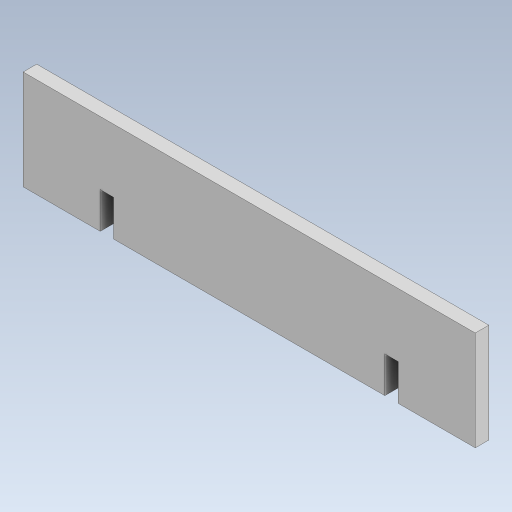
# Autodesk Inventor part: 零件8
Saved by Autodesk Inventor 2023 (Build 270158000, 158)
## iProperties
Created: 2023-05-16
Part Number: 零件8
Material: 一般
Document SubType Name: Modeling
Designer: Johnny Jou
Density: 1 g/cm^3
Appearance: 預設
Author: Johnny Jou
Autodesk Inventor part; units mm, degrees
ref_plane "YZ Plane" through (0, 0, 0) normal (1, 0, 0) x (0, 1, 0)
ref_plane "XZ Plane" through (0, 0, 0) normal (0, 1, 0) x (-1, 0, 0)
ref_plane "XY Plane" through (0, 0, 0) normal (0, 0, 1) x (1, 0, 0)
sketch "草圖1" plane through (0, 0, 0) normal (0, 0, 1) x (1, 0, 0)
  line L0 (0, 0) -> (100, 0)
  line L1 (100, 0) -> (100, -22)
  line L2 (100, -22) -> (0, -22)
  line L3 (0, -22) -> (0, 0)
  line L4 (17.05, -22) -> (20, -22)
  line L5 (20, -22) -> (20, -14)
  line L6 (20, -14) -> (17.05, -14)
  line L7 (17.05, -14) -> (17.05, -22)
  line L8 (80, -22) -> (82.95, -22)
  line L9 (82.95, -22) -> (82.95, -14)
  line L10 (82.95, -14) -> (80, -14)
  line L11 (80, -14) -> (80, -22)
  line L12 (20, -14) -> (80, -14)
  point P0 (50, -14)
  point P1 (50, -22)
  dimension "d0" = 60
  dimension "d1" = 100
  dimension "d2" = 2.95
  dimension "d3" = 2.95
  dimension "d4" = 8
  dimension "d5" = 22
  constraints: 26 end point, 6 parallel, 4 perpendicular, 4 point on line, 2 midpoint, 1 horizontal, 1 vertical alignment
  measures "d0" distance between parallel lines of L11 L5
  measures "d1" distance of L1.end L2.end
  measures "d2" distance of L9.end L10.end
  measures "d3" distance of L5.end L6.end
  measures "d4" distance of L6.end L4.start
  measures "d5" distance of L0.end L1.end
extrude "擠出1" add sketch "草圖1" along normal blind 3 contours L0 L1 L2 L9 L10 L12 L6 L7 L3 | L5 L12 L11 L2
